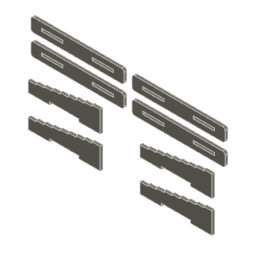
cut 4 (Autodesk Fusion 360 design; units mm, degrees)
part number: 2026-03-12-17-42-55-001
Autodesk Fusion 360 part; units mm, degrees
sketch "cart blocks multiple" plane through (0, 0, 0) normal (0, 0, 1) x (1, 0, 0)
  line L0 (304.8, 41.275) -> (323.85, 41.275)
  line L1 (228.6, 28.575) -> (247.65, 28.575)
  line L2 (342.9, 47.625) -> (361.95, 47.625)
  line L3 (247.65, 28.575) -> (247.65, 31.75)
  line L4 (209.55, 0) -> (209.55, 25.4)
  line L5 (266.7, 31.75) -> (266.7, 34.925)
  line L6 (209.55, 25.4) -> (228.6, 25.4)
  line L7 (285.75, 38.1) -> (304.8, 38.1)
  line L8 (304.8, 38.1) -> (304.8, 41.275)
  line L9 (247.65, 31.75) -> (266.7, 31.75)
  line L10 (228.6, 25.4) -> (228.6, 28.575)
  line L11 (342.9, 44.45) -> (342.9, 47.625)
  line L12 (323.85, 44.45) -> (342.9, 44.45)
  line L13 (323.85, 41.275) -> (323.85, 44.45)
  line L14 (260.35, 6.35) -> (260.35, 0)
  line L15 (266.7, 34.925) -> (285.75, 34.925)
  line L16 (285.75, 34.925) -> (285.75, 38.1)
  line L17 (381, 0) -> (330.2, 0)
  line L18 (260.35, 0) -> (209.55, 0)
  line L19 (361.95, 47.625) -> (361.95, 50.8)
  line L20 (330.2, 6.35) -> (260.35, 6.35)
  line L21 (381, 50.8) -> (381, 0)
  line L22 (330.2, 0) -> (330.2, 6.35)
  line L23 (361.95, 50.8) -> (381, 50.8)
  line L24 (57.15, 31.75) -> (57.15, 34.925)
  line L25 (95.25, 41.275) -> (114.3, 41.275)
  line L26 (114.3, 44.45) -> (133.35, 44.45)
  line L27 (171.45, 0) -> (120.65, 0)
  line L28 (76.2, 38.1) -> (95.25, 38.1)
  line L29 (152.4, 47.625) -> (152.4, 50.8)
  line L30 (50.8, 6.35) -> (50.8, 0)
  line L31 (38.1, 28.575) -> (38.1, 31.75)
  line L32 (38.1, 31.75) -> (57.15, 31.75)
  line L33 (19.05, 25.4) -> (19.05, 28.575)
  line L34 (133.35, 44.45) -> (133.35, 47.625)
  line L35 (120.65, 6.35) -> (50.8, 6.35)
  line L36 (120.65, 0) -> (120.65, 6.35)
  line L37 (171.45, 50.8) -> (171.45, 0)
  line L38 (152.4, 50.8) -> (171.45, 50.8)
  line L39 (19.05, 28.575) -> (38.1, 28.575)
  line L40 (95.25, 38.1) -> (95.25, 41.275)
  line L41 (0, 25.4) -> (19.05, 25.4)
  line L42 (50.8, 0) -> (0, 0)
  line L43 (133.35, 47.625) -> (152.4, 47.625)
  line L44 (114.3, 41.275) -> (114.3, 44.45)
  line L45 (0, 0) -> (0, 25.4)
  line L46 (76.2, 34.925) -> (76.2, 38.1)
  line L47 (57.15, 34.925) -> (76.2, 34.925)
  line L48 (152.4, 123.825) -> (152.4, 127)
  line L49 (133.35, 120.65) -> (133.35, 123.825)
  line L50 (50.8, 76.2) -> (0, 76.2)
  line L51 (38.1, 104.775) -> (38.1, 107.95)
  line L52 (76.2, 111.125) -> (76.2, 114.3)
  line L53 (57.15, 107.95) -> (57.15, 111.125)
  line L54 (171.45, 127) -> (171.45, 76.2)
  line L55 (95.25, 117.475) -> (114.3, 117.475)
  line L56 (19.05, 101.6) -> (19.05, 104.775)
  line L57 (76.2, 114.3) -> (95.25, 114.3)
  line L58 (133.35, 123.825) -> (152.4, 123.825)
  line L59 (95.25, 114.3) -> (95.25, 117.475)
  line L60 (38.1, 107.95) -> (57.15, 107.95)
  line L61 (57.15, 111.125) -> (76.2, 111.125)
  line L62 (19.05, 104.775) -> (38.1, 104.775)
  line L63 (114.3, 120.65) -> (133.35, 120.65)
  line L64 (171.45, 76.2) -> (120.65, 76.2)
  line L65 (120.65, 76.2) -> (120.65, 82.55)
  line L66 (0, 76.2) -> (0, 101.6)
  line L67 (114.3, 117.475) -> (114.3, 120.65)
  line L68 (152.4, 127) -> (171.45, 127)
  line L69 (0, 101.6) -> (19.05, 101.6)
  line L70 (50.8, 82.55) -> (50.8, 76.2)
  line L71 (120.65, 82.55) -> (50.8, 82.55)
  line L72 (323.85, 117.475) -> (323.85, 120.65)
  line L73 (381, 127) -> (381, 76.2)
  line L74 (209.55, 101.6) -> (228.6, 101.6)
  line L75 (247.65, 107.95) -> (266.7, 107.95)
  line L76 (381, 76.2) -> (330.2, 76.2)
  line L77 (266.7, 111.125) -> (285.75, 111.125)
  line L78 (285.75, 111.125) -> (285.75, 114.3)
  line L79 (323.85, 120.65) -> (342.9, 120.65)
  line L80 (361.95, 127) -> (381, 127)
  line L81 (361.95, 123.825) -> (361.95, 127)
  line L82 (330.2, 82.55) -> (260.35, 82.55)
  line L83 (342.9, 123.825) -> (361.95, 123.825)
  line L84 (266.7, 107.95) -> (266.7, 111.125)
  line L85 (304.8, 117.475) -> (323.85, 117.475)
  line L86 (260.35, 82.55) -> (260.35, 76.2)
  line L87 (260.35, 76.2) -> (209.55, 76.2)
  line L88 (228.6, 101.6) -> (228.6, 104.775)
  line L89 (285.75, 114.3) -> (304.8, 114.3)
  line L90 (304.8, 114.3) -> (304.8, 117.475)
  line L91 (247.65, 104.775) -> (247.65, 107.95)
  line L92 (330.2, 76.2) -> (330.2, 82.55)
  line L93 (342.9, 120.65) -> (342.9, 123.825)
  line L94 (228.6, 104.775) -> (247.65, 104.775)
  line L95 (209.55, 76.2) -> (209.55, 101.6)
  line L96 (215.9838, 146.05) -> (6.3796, 146.05)
  spline S0 degree 3 poles (6.3796, 146.05) (2.8563, 146.05) (0, 148.9063) (0, 152.4296) knots 1 1 1 1 2 2 2 2
  line L97 (0, 152.4296) -> (0, 171.4926)
  spline S1 degree 3 poles (0, 171.4926) (0, 174.9761) (2.8239, 177.8) (6.3074, 177.8) knots 3 3 3 3 4 4 4 4
  line L98 (6.3074, 177.8) -> (215.9287, 177.8)
  spline S2 degree 3 poles (215.9287, 177.8) (219.4199, 177.8) (222.25, 174.9699) (222.25, 171.4787) knots 5 5 5 5 6 6 6 6
  line L99 (222.25, 171.4787) -> (222.25, 152.3162)
  spline S3 degree 3 poles (222.25, 152.3162) (222.25, 148.8555) (219.4445, 146.05) (215.9838, 146.05) knots 7 7 7 7 8 8 8 8
  line L100 (76.2, 165.1) -> (76.2, 158.7501)
  line L101 (25.4, 158.7501) -> (25.4, 165.1)
  line L102 (25.4, 165.1) -> (76.2, 165.1)
  line L103 (76.2, 158.7501) -> (25.4, 158.7501)
  line L104 (146.05, 158.7501) -> (146.05, 165.1)
  line L105 (146.05, 165.1) -> (196.85, 165.1)
  line L106 (196.85, 158.7501) -> (146.05, 158.7501)
  line L107 (196.85, 165.1) -> (196.85, 158.7501)
  line L108 (450.9338, 146.05) -> (241.3296, 146.05)
  spline S4 degree 3 poles (241.3296, 146.05) (237.8063, 146.05) (234.95, 148.9063) (234.95, 152.4296) knots 1 1 1 1 2 2 2 2
  line L109 (234.95, 152.4296) -> (234.95, 171.4926)
  spline S5 degree 3 poles (234.95, 171.4926) (234.95, 174.9761) (237.7739, 177.8) (241.2574, 177.8) knots 3 3 3 3 4 4 4 4
  line L110 (241.2574, 177.8) -> (450.8787, 177.8)
  spline S6 degree 3 poles (450.8787, 177.8) (454.3699, 177.8) (457.2, 174.9699) (457.2, 171.4787) knots 5 5 5 5 6 6 6 6
  line L111 (457.2, 171.4787) -> (457.2, 152.3162)
  spline S7 degree 3 poles (457.2, 152.3162) (457.2, 148.8555) (454.3945, 146.05) (450.9338, 146.05) knots 7 7 7 7 8 8 8 8
  line L112 (260.35, 158.7501) -> (260.35, 165.1)
  line L113 (311.15, 165.1) -> (311.15, 158.7501)
  line L114 (260.35, 165.1) -> (311.15, 165.1)
  line L115 (311.15, 158.7501) -> (260.35, 158.7501)
  line L116 (431.8, 158.7501) -> (381, 158.7501)
  line L117 (431.8, 165.1) -> (431.8, 158.7501)
  line L118 (381, 158.7501) -> (381, 165.1)
  line L119 (381, 165.1) -> (431.8, 165.1)
  line L120 (450.9338, 196.85) -> (241.3296, 196.85)
  spline S8 degree 3 poles (241.3296, 196.85) (237.8063, 196.85) (234.95, 199.7063) (234.95, 203.2296) knots 1 1 1 1 2 2 2 2
  line L121 (234.95, 203.2296) -> (234.95, 222.2926)
  spline S9 degree 3 poles (234.95, 222.2926) (234.95, 225.7761) (237.7739, 228.6) (241.2574, 228.6) knots 3 3 3 3 4 4 4 4
  line L122 (241.2574, 228.6) -> (450.8787, 228.6)
  spline S10 degree 3 poles (450.8787, 228.6) (454.3699, 228.6) (457.2, 225.7699) (457.2, 222.2787) knots 5 5 5 5 6 6 6 6
  line L123 (457.2, 222.2787) -> (457.2, 203.1162)
  spline S11 degree 3 poles (457.2, 203.1162) (457.2, 199.6555) (454.3945, 196.85) (450.9338, 196.85) knots 7 7 7 7 8 8 8 8
  line L124 (311.15, 209.5501) -> (260.35, 209.5501)
  line L125 (311.15, 215.9) -> (311.15, 209.5501)
  line L126 (260.35, 209.5501) -> (260.35, 215.9)
  line L127 (260.35, 215.9) -> (311.15, 215.9)
  line L128 (431.8, 209.5501) -> (381, 209.5501)
  line L129 (381, 209.5501) -> (381, 215.9)
  line L130 (431.8, 215.9) -> (431.8, 209.5501)
  line L131 (381, 215.9) -> (431.8, 215.9)
  line L132 (215.9838, 196.85) -> (6.3796, 196.85)
  spline S12 degree 3 poles (6.3796, 196.85) (2.8563, 196.85) (0, 199.7063) (0, 203.2296) knots 1 1 1 1 2 2 2 2
  line L133 (0, 203.2296) -> (0, 222.2926)
  spline S13 degree 3 poles (0, 222.2926) (0, 225.7761) (2.8239, 228.6) (6.3074, 228.6) knots 3 3 3 3 4 4 4 4
  line L134 (6.3074, 228.6) -> (215.9287, 228.6)
  spline S14 degree 3 poles (215.9287, 228.6) (219.4199, 228.6) (222.25, 225.7699) (222.25, 222.2787) knots 5 5 5 5 6 6 6 6
  line L135 (222.25, 222.2787) -> (222.25, 203.1162)
  spline S15 degree 3 poles (222.25, 203.1162) (222.25, 199.6555) (219.4445, 196.85) (215.9838, 196.85) knots 7 7 7 7 8 8 8 8
  line L136 (25.4, 215.9) -> (76.2, 215.9)
  line L137 (25.4, 209.5501) -> (25.4, 215.9)
  line L138 (76.2, 215.9) -> (76.2, 209.5501)
  line L139 (76.2, 209.5501) -> (25.4, 209.5501)
  line L140 (196.85, 209.5501) -> (146.05, 209.5501)
  line L141 (196.85, 215.9) -> (196.85, 209.5501)
  line L142 (146.05, 215.9) -> (196.85, 215.9)
  line L143 (146.05, 209.5501) -> (146.05, 215.9)
sketch "cart block base" plane through (0, 0, 0) normal (0, 0, 1) x (1, 0, 0)
  line L0 (212.8088, -155.7514) -> (3.2046, -155.7514)
  spline S0 degree 3 poles (3.2046, -155.7514) (-0.3187, -155.7514) (-3.175, -152.8951) (-3.175, -149.3718) knots 1 1 1 1 2 2 2 2
  line L1 (-3.175, -149.3718) -> (-3.175, -130.3088)
  spline S1 degree 3 poles (-3.175, -130.3088) (-3.175, -126.8253) (-0.3511, -124.0014) (3.1324, -124.0014) knots 3 3 3 3 4 4 4 4
  line L2 (3.1324, -124.0014) -> (212.7537, -124.0014)
  spline S2 degree 3 poles (212.7537, -124.0014) (216.2449, -124.0014) (219.075, -126.8315) (219.075, -130.3227) knots 5 5 5 5 6 6 6 6
  line L3 (219.075, -130.3227) -> (219.075, -149.4852)
  spline S3 degree 3 poles (219.075, -149.4852) (219.075, -152.9459) (216.2695, -155.7514) (212.8088, -155.7514) knots 7 7 7 7 8 8 8 8
  line L4 (22.225, -143.0512) -> (22.225, -136.7014)
  line L5 (73.025, -143.0512) -> (22.225, -143.0512)
  line L6 (22.225, -136.7014) -> (73.025, -136.7014)
  line L7 (73.025, -136.7014) -> (73.025, -143.0512)
  line L8 (193.675, -143.0512) -> (142.875, -143.0512)
  line L9 (193.675, -136.7014) -> (193.675, -143.0512)
  line L10 (142.875, -136.7014) -> (193.675, -136.7014)
  line L11 (142.875, -143.0512) -> (142.875, -136.7014)
extrude "Extrude2" add sketch "cart block base" along normal blind 6.35 makes body 1
move_body "Move1" bodies 1 to x (1, 0, 0) y (0, 1, 0) z (0, 0, 1) at (0, 330.2, 0)
copy_body "CopyPasteBodies1" bodies 1 makes body 2
move_body "Move2" bodies 2 to x (1, 0, 0) y (0, 1, 0) z (0, 0, 1) at (254, 0, 0)
copy_body "CopyPasteBodies2" bodies 2 makes body 3
move_body "Move3" bodies 3 to x (1, 0, 0) y (0, 1, 0) z (0, 0, 1) at (0, 50.8, 0)
copy_body "CopyPasteBodies3" bodies 3 makes body 4
move_body "Move4" bodies 4 to x (1, 0, 0) y (0, 1, 0) z (0, 0, 1) at (-254, 0, 0)
sketch "cart block holder" plane through (0, 0, 0) normal (0, 0, 1) x (1, 0, 0)
  line L0 (136.5175, 63.3799) -> (136.5175, 66.5549)
  line L1 (98.4175, 57.0299) -> (98.4175, 60.2049)
  line L2 (60.3175, 50.6799) -> (60.3175, 53.8549)
  line L3 (117.4675, 63.3799) -> (136.5175, 63.3799)
  line L4 (155.5675, 69.7299) -> (174.6175, 69.7299)
  line L5 (174.6175, 69.7299) -> (174.6175, 18.9299)
  line L6 (53.9675, 18.9299) -> (3.1675, 18.9299)
  line L7 (53.9675, 25.2799) -> (53.9675, 18.9299)
  line L8 (60.3175, 53.8549) -> (79.3675, 53.8549)
  line L9 (79.3675, 53.8549) -> (79.3675, 57.0299)
  line L10 (98.4175, 60.2049) -> (117.4675, 60.2049)
  line L11 (123.8175, 25.2799) -> (53.9675, 25.2799)
  line L12 (79.3675, 57.0299) -> (98.4175, 57.0299)
  line L13 (136.5175, 66.5549) -> (155.5675, 66.5549)
  line L14 (174.6175, 18.9299) -> (123.8175, 18.9299)
  line L15 (3.1675, 18.9299) -> (3.1675, 44.3299)
  line L16 (117.4675, 60.2049) -> (117.4675, 63.3799)
  line L17 (22.2175, 47.5049) -> (41.2675, 47.5049)
  line L18 (41.2675, 50.6799) -> (60.3175, 50.6799)
  line L19 (3.1675, 44.3299) -> (22.2175, 44.3299)
  line L20 (22.2175, 44.3299) -> (22.2175, 47.5049)
  line L21 (41.2675, 47.5049) -> (41.2675, 50.6799)
  line L22 (155.5675, 66.5549) -> (155.5675, 69.7299)
  line L23 (123.8175, 18.9299) -> (123.8175, 25.2799)
extrude "Extrude3" add sketch "cart block holder" along normal blind 6.35 separate body makes body 5
copy_body "CopyPasteBodies4" bodies 5 makes body 6
move_body "Move5" bodies 6 to x (1, 0, 0) y (0, 1, 0) z (0, 0, 1) at (266.7, 0, 0)
copy_body "CopyPasteBodies5" bodies 6 makes body 7
move_body "Move6" bodies 7 to x (1, 0, 0) y (0, 1, 0) z (0, 0, 1) at (0, 76.2, 0)
copy_body "CopyPasteBodies6" bodies 7 makes body 8
move_body "Move7" bodies 8 to x (1, 0, 0) y (0, 1, 0) z (0, 0, 1) at (-266.7, 0, 0)
move_body "Move8" bodies 4 to x (1, 0, 0) y (0, 1, 0) z (0, 0, 1) at (12.7, 0, 0)
move_body "Move9" bodies 1 to x (1, 0, 0) y (0, 1, 0) z (0, 0, 1) at (12.7, 0, 0)
